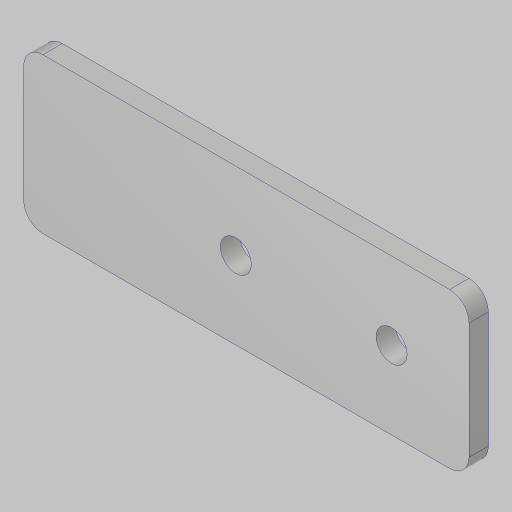
# Autodesk Inventor part: EL2-016
Saved by Autodesk Inventor 2023.5 (Build 275446000, 446)
## iProperties
Created: 2025-01-21
Part Number: EL2-016
Material: Aluminum 6061
Document SubType Name: Modeling
Designer: slick
Density: 2.7 g/cm^3
Appearance: Aluminum - Flat
Author: slick
Autodesk Inventor part; units mm, degrees
ref_plane "YZ Plane" through (0, 0, 0) normal (1, 0, 0) x (0, 1, 0)
ref_plane "XZ Plane" through (0, 0, 0) normal (0, 1, 0) x (-1, 0, 0)
ref_plane "XY Plane" through (0, 0, 0) normal (0, 0, 1) x (1, 0, 0)
sketch "Sketch1" plane through (0, 0, 0) normal (0, 0, 1) x (1, 0, 0)
  line L0 (-36.5125, 12.7) -> (36.5125, 12.7)
  line L1 (36.5125, 12.7) -> (36.5125, -12.7)
  line L2 (36.5125, -12.7) -> (-36.5125, -12.7)
  line L3 (-36.5125, -12.7) -> (-36.5125, 12.7)
  line L4 (-36.5125, 12.7) -> (36.5125, -12.7) construction
  line L5 (36.5125, 12.7) -> (-36.5125, -12.7) construction
  point P0 (0, 0)
  dimension "d15" = 73.025
  dimension "d16" = 25.4
  constraints: 12 end point, 2 midpoint, 2 parallel, 1 horizontal, 1 perpendicular
  measures "d15" distance of L1.end L2.end
  measures "d16" distance of L0.end L1.end
extrude "Extrusion1" add sketch "Sketch1" along normal blind 3.175
sketch "Sketch3" plane through (0, 0, 3.175) normal (0, 0, 1) x (1, 0, 0)
  line L0 (-36.5125, 12.7) -> (-36.5125, -12.7) projected
  line L1 (36.5125, -12.7) -> (36.5125, 12.7) projected
  point P0 (0, 0)
  point P1 (23.8125, 0)
  point P2 (-1.7145, 0)
  point P3 (36.5125, 0)
  dimension "d17" = 25.527
  dimension "d27" = 12.7
  constraints: 2 horizontal alignment, 1 midpoint
  measures "d17" distance of point (23.812, 0) point (-1.714, 0)
  measures "d27" distance of point (36.513, 0) point (23.812, 0)
hole "Hole2" at (23.8125, 0, 3.175) at (-1.7145, 0, 3.175) direction (0, 0, -1) diameter 5.1054 end through all clearance for "Flat Head Machine Screw (82)" size "#10" standard "Ansi Unified Screw Threads"
fillet "Fillet2" radius 3.175 4 edges at (-36.5125, 12.7, 1.5875) (-36.5125, -12.7, 1.5875) (36.5125, 12.7, 1.5875) (36.5125, -12.7, 1.5875)
body "Solid1"
